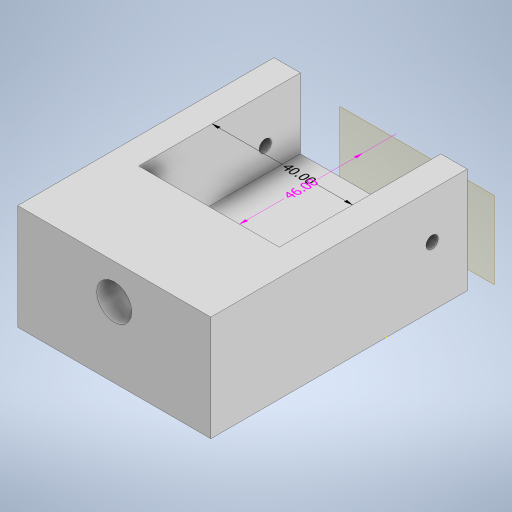
# Autodesk Inventor part: camera_support_2
Saved by Autodesk Inventor 2023 (Build 270158000, 158)
## iProperties
Created: 2022-07-04
Part Number: camera_support_2
Material: Genérico
Document SubType Name: Modeling
Designer: inigo
Density: 1 g/cm^3
Appearance: Valor por defecto
Author: inigo
Autodesk Inventor part; units mm, degrees
ref_plane "YZ Plane" through (0, 0, 0) normal (1, 0, 0) x (0, 1, 0)
ref_plane "XZ Plane" through (0, 0, 0) normal (0, 1, 0) x (-1, 0, 0)
ref_plane "XY Plane" through (0, 0, 0) normal (0, 0, 1) x (1, 0, 0)
sketch "Boceto1" plane through (0, 0, 0) normal (0, 1, 0) x (-1, 0, 0)
  line L0 (27.5, 50) -> (-27.5, 50)
  line L1 (-27.5, 50) -> (-27.5, -50)
  line L2 (-27.5, -50) -> (27.5, -50)
  line L3 (27.5, -50) -> (27.5, 50)
  line L4 (27.5, 50) -> (-27.5, -50) construction
  line L5 (-27.5, 50) -> (27.5, -50) construction
  point P0 (0, 0)
  dimension "d0" = 55
  dimension "d1" = 100
  constraints: 12 end point, 2 midpoint, 2 parallel, 1 horizontal, 1 perpendicular
  measures "d0" distance of L2.end L1.end
  measures "d1" distance of L1.end L0.end
extrude "Extrusión1" add sketch "Boceto1" along normal blind 30
sketch "Boceto2" plane through (27.5, 0, -50) normal (0, 0, -1) x (-1, 0, 0)
  line L0 (22.5, 25) -> (32.5, 25)
  line L1 (32.5, 25) -> (32.5, 5)
  line L2 (32.5, 5) -> (22.5, 5)
  line L3 (22.5, 5) -> (22.5, 25)
  line L4 (22.5, 25) -> (32.5, 5) construction
  line L5 (32.5, 25) -> (22.5, 5) construction
  line L6 (0, 30) -> (55, 30) projected
  line L7 (0, 0) -> (0, 30) projected
  line L8 (55, 0) -> (55, 30) projected
  point P0 (27.5, 0)
  point P1 (27.5, 15)
  point P2 (27.5, 25)
  dimension "d4" = 10
  dimension "d5" = 20
  dimension "d6" = 5
  dimension "d7" = 22.5
  dimension "d24" = 22.5
  constraints: 12 end point, 3 midpoint, 2 parallel, 1 horizontal, 1 perpendicular
  measures "d4" distance of L1.end L2.end
  measures "d5" distance of L0.end L1.end
  measures "d6" distance from line of L6 point (27.5, 25)
  measures "d7" distance between parallel lines of L3 L7
  measures "d24" distance between parallel lines of L8 L1
extrude "Extrusión2" add sketch "Boceto2" along normal blind 10
sketch "Boceto3" plane through (-27.5, 0, 50) normal (0, 0, 1) x (1, 0, 0)
  circle A0 centre (27.5, 20) radius 5
  line L0 (0, 30) -> (55, 30) projected
  point P0 (27.5, 0)
  point P1 (27.5, 30)
  dimension "d10" = 10
  dimension "d11" = 10
  constraints: 1 centre point, 1 midpoint
  measures "d10" diameter of A0
  measures "d11" distance of point (27.5, 30) A0.centre
extrude "Extrusión3" cut sketch "Boceto3" against normal blind 15
sketch "Boceto4" plane through (0, 30, 0) normal (0, 1, 0) x (1, 0, 0)
  line L0 (-20, 23) -> (20, 23)
  line L1 (20, 23) -> (20, -23)
  line L2 (20, -23) -> (-20, -23)
  line L3 (-20, -23) -> (-20, 23)
  line L4 (-20, 23) -> (20, -23) construction
  line L5 (20, 23) -> (-20, -23) construction
  point P0 (0, 0)
  dimension "d14" = 40
  dimension "d15" = 46
  constraints: 12 end point, 2 midpoint, 2 parallel, 1 horizontal, 1 perpendicular
  measures "d14" distance of L1.end L2.end
  measures "d15" distance of L0.end L1.end
extrude "Extrusión4" cut sketch "Boceto4" against normal blind 20
ref_plane "Plano de trabajo1" through (0, 5, -50) normal (1, 0, 0) x (0, 0, -1)
sketch "Boceto5" plane through (0, 5, -50) normal (1, 0, 0) x (0, 0, -1)
  line L0 (7.5, 0) -> (0, -2.5)
  line L1 (0, -2.5) -> (0, 0)
  line L2 (0, 0) -> (7.5, 0)
  point P0 (-50, -5)
  point P1 (0, -5)
  point P2 (10, 0)
  dimension "d25" = 2.5
  dimension "d26" = 2.5
  constraints: 6 end point
  measures "d25" distance of point (0, -5) L0.end
  measures "d26" distance of point (10, 0) L0.start
extrude "Extrusión5" add sketch "Boceto5" along normal mid plane 8
ref_plane "Plano de trabajo2" through (0, 15, 0) normal (0, -1, 0) x (1, 0, 0)
sketch "Boceto6" plane through (0, 15, 0) normal (0, -1, 0) x (1, 0, 0)
  line L0 (5, -50) -> (8, -50)
  line L1 (27.5, -50) -> (-27.5, -50)
  line L2 (5, -57) -> (8, -50)
  line L3 (4, -50) -> (5, -50) projected
  line L4 (5, -50) -> (5, -57)
  line L5 (0, -50.2371) -> (0, -56.5746)
  line L6 (-5, -50) -> (-8, -50)
  line L7 (-27.5, -50) -> (27.5, -50)
  line L8 (-5, -57) -> (-8, -50)
  line L9 (-4, -50) -> (-5, -50)
  line L10 (-5, -50) -> (-5, -57)
  point P0 (0, 0)
  point P1 (5, -60)
  point P2 (-5, -60)
  dimension "d29" = 3
  dimension "d30" = 3
  constraints: 20 end point, 7 symmetric about line, 2 point on line, 1 vertical
  measures "d29" distance of L0.start L0.end
  measures "d30" distance of point (5, -60) L2.start
extrude "Extrusión6" add sketch "Boceto6" along normal mid plane 8
sketch "Boceto7" plane through (27.5, 0, 50) normal (1, 0, 0) x (0, 0, -1)
  point P0 (50, 0)
ref_plane "Plano de trabajo4" through (-20, 30, -23) normal (0, 0, 1) x (1, 0, 0)
sketch "Boceto8" plane through (27.5, 0, 50) normal (1, 0, 0) x (0, 0, -1)
  line L0 (58, 22) -> (88, 22)
  circle A0 centre (83, 17) radius 1.75
  line L1 (63, 17) -> (83, 17)
  line L2 (88, 22) -> (88, 12)
  circle A1 centre (63, 17) radius 1.75
  line L3 (58, 12) -> (88, 22) construction
  line L4 (58, 22) -> (88, 12) construction
  line L5 (58, 12) -> (58, 22)
  line L6 (88, 12) -> (58, 12)
  line L7 (73, 30) -> (73, 10) projected
  line L8 (0, 30) -> (100, 30) projected
  point P0 (50, 0)
  point P1 (72.9522, 12.5553)
  point P2 (57.9522, 14.5161)
  point P3 (72.9522, 12.5553)
  point P4 (88, 17)
  dimension "d34" = 10
  dimension "d35" = 30
  dimension "d36" = 5
  dimension "d37" = 5
  dimension "d38" = 5
  dimension "d39" = 5
  dimension "d40" = 10
  dimension "d41" = 8
  constraints: 6 end point, 2 centre point, 1 midpoint, 12 other
  measures "d34" distance between parallel lines of L6 L0
  measures "d36" distance of point (88, 17) A0.centre
  measures "d37" distance from line of L0 A0.centre
  measures "d38" distance from line of L0 A1.centre
  measures "d40" distance from line of L7 A0.centre
  measures "d41" distance between parallel lines of L8 L0
hole "Agujero1" at (27.5, 17, -13) at (27.5, 17, -33) direction (-1, 0, 0) diameter 3.5 end through all
split "Dividir1" plane through (-20, 30, -23) removes the side toward (0, 0, -1)
